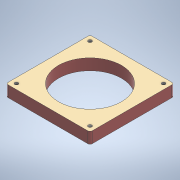
# Autodesk Inventor part: NoctuaNF-A12x15
Saved by Autodesk Inventor 2020 (Build 240168000, 168)
## iProperties
Created: 2020-04-06
Part Number: NoctuaNF-A12x15
Material: Типовые
Document SubType Name: Modeling
Designer: Михаил
Density: 1 g/cm^3
Appearance: По умолчанию
Author: Михаил
Autodesk Inventor part; units mm, degrees
ref_plane "YZ Plane" through (0, 0, 0) normal (1, 0, 0) x (0, 1, 0)
ref_plane "XZ Plane" through (0, 0, 0) normal (0, 1, 0) x (-1, 0, 0)
ref_plane "XY Plane" through (0, 0, 0) normal (0, 0, 1) x (1, 0, 0)
sketch "Эскиз1" plane through (0, 0, 0) normal (0, 1, 0) x (-1, 0, 0)
  line L0 (0, 0) -> (120, 0)
  line L1 (120, 0) -> (120, -120)
  line L2 (120, -120) -> (0, -120)
  line L3 (0, -120) -> (0, 0)
  dimension "d0" = 120
  dimension "d1" = 120
  constraints: 8 end point, 2 parallel, 1 horizontal, 1 perpendicular
  measures "d0" distance of L1.end L2.end
  measures "d1" distance of L0.end L1.end
sketch "Эскиз2" plane through (0, 0, 0) normal (0, 1, 0) x (-1, 0, 0)
  circle A0 centre (60, -60) radius 45
  point P0 (0, 0)
  dimension "d2" = 90
  dimension "d3" = 60
  dimension "d4" = 60
  constraints: 1 centre point
  measures "d2" diameter of A0
  measures "d3" horizontal distance of point (0, 0) A0.centre
  measures "d4" horizontal distance of point (0, 0) A0.centre
extrude "Выдавливание1" add sketch "Эскиз1" along normal blind 16
fillet "Сопряжение1" radius 3 4 edges at (-120, 8, 0) (0, 8, 0) (0, 8, -120) (-120, 8, -120)
extrude "Выдавливание2" cut sketch "Эскиз2" along normal blind 16
sketch "Эскиз3" plane through (0, 16, 0) normal (0, 1, 0) x (1, 0, 0)
  circle A0 centre (-112.5, 7.5) radius 2.5
  circle A1 centre (-7.5, 7.5) radius 2.5
  circle A2 centre (-7.5, 112.5) radius 2.5
  circle A3 centre (-112.5, 112.5) radius 2.5
  line L0 (0, 3) -> (0, 117) projected
  point P0 (0, 0)
  dimension "d10" = 5
  dimension "d11" = 5
  dimension "d12" = 5
  dimension "d13" = 5
  dimension "d14" = 112.5
  dimension "d15" = 7.5
  dimension "d16" = 7.5
  dimension "d17" = 7.5
  dimension "d18" = 105
  dimension "d19" = 7.5
  dimension "d20" = 105
  dimension "d21" = 105
  constraints: 4 centre point
  measures "d10" diameter of A0
  measures "d11" diameter of A1
  measures "d12" diameter of A2
  measures "d13" diameter of A3
  measures "d14" horizontal distance of point (0, 0) A0.centre
  measures "d15" vertical distance of point (0, 0) A0.centre
  measures "d16" horizontal distance of point (0, 0) A1.centre
  measures "d17" horizontal distance of point (0, 0) A1.centre
  measures "d18" distance of A1.centre A2.centre
  measures "d19" distance from line of L0 A2.centre
  measures "d20" distance of A3.centre A2.centre
  measures "d21" distance of A0.centre A3.centre
extrude "Выдавливание3" cut sketch "Эскиз3" against normal blind 16
